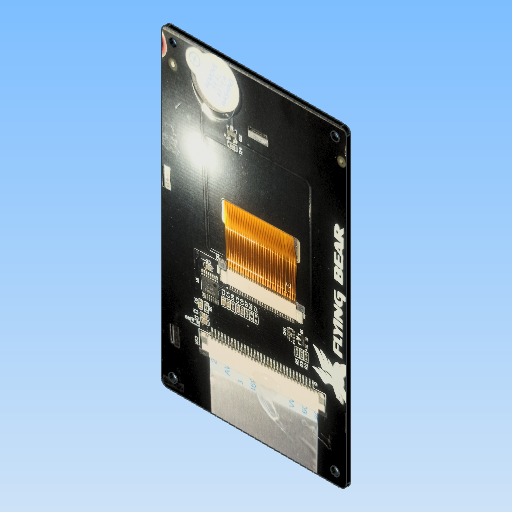
# Autodesk Inventor part: ЭКРАН
Saved by Autodesk Inventor 2017 (Build 210142000, 142)
## iProperties
Part Number: ЭКРАН
Material: Типовые
Document SubType Name: Modeling
Designer: Max
Mass: 9.96561 g
Surface Area: 147.746 cm^2
Volume: 9.96561 cm^3
Density: 1 g/cm^3
Appearance: Оружейный металл — полированный
Author: Max
Autodesk Inventor part; units mm, degrees
ref_plane "YZ Plane" through (0, 0, 0) normal (1, 0, 0) x (0, 1, 0)
ref_plane "XZ Plane" through (0, 0, 0) normal (0, 1, 0) x (-1, 0, 0)
ref_plane "XY Plane" through (0, 0, 0) normal (0, 0, 1) x (1, 0, 0)
sketch "Эскиз1" plane through (0, 0, 0) normal (0, 0, 1) x (1, 0, 0)
  line L0 (28.5, 51) -> (-28.5, 51) construction
  line L1 (-28.5, 51) -> (-28.5, -51) construction
  line L2 (-28.5, -51) -> (28.5, -51) construction
  line L3 (28.5, -51) -> (28.5, 51) construction
  line L4 (28.5, 51) -> (-28.5, -51) construction
  line L5 (-28.5, 51) -> (28.5, -51) construction
  circle A0 centre (-28.5, 51) radius 1.5
  circle A1 centre (28.5, 51) radius 1.5
  circle A2 centre (-28.5, -51) radius 1.5
  circle A3 centre (28.5, -51) radius 1.5
  line L6 (32.5, -55) -> (-32.5, -55)
  line L7 (-32.5, -55) -> (-32.5, 55)
  line L8 (-32.5, 55) -> (32.5, 55)
  line L9 (32.5, 55) -> (32.5, -55)
  line L10 (32.5, -55) -> (-32.5, 55) construction
  line L11 (-32.5, -55) -> (32.5, 55) construction
  point P0 (0, 0)
  point P1 (0, 0)
  dimension "d0" = 57
  dimension "d1" = 102
  dimension "d2" = 3
  dimension "d3" = 3
  dimension "d4" = 3
  dimension "d5" = 3
  dimension "d6" = 65
  dimension "d7" = 110
  constraints: 24 end point, 6 midpoint, 4 centre point, 4 coincident, 4 parallel, 2 horizontal, 2 perpendicular
  measures "d0" distance of L2.end L1.end
  measures "d1" distance of L1.end L0.end
  measures "d2" diameter of A0
  measures "d3" diameter of A1
  measures "d4" diameter of A2
  measures "d5" diameter of A3
  measures "d6" distance between parallel lines of L9 L7
  measures "d7" distance between parallel lines of L6 L8
extrude "Выдавливание1" add sketch "Эскиз1" along normal blind 1.4
fillet "Сопряжение1" radius 2 4 edges at (-32.5, 55, 0.7) (32.5, 55, 0.7) (-32.5, -55, 0.7) (32.5, -55, 0.7)
sketch "Эскиз2" plane through (0, 0, 1.4) normal (0, 0, 1) x (1, 0, 0)
  line L0 (36.1838, 87.7862) -> (49.9544, -99.5548) construction
  line L1 (49.9544, -99.5548) -> (-36.5855, -105.916) construction
  line L2 (-36.5855, -105.916) -> (-50.3561, 81.4251) construction
  line L3 (-50.3561, 81.4251) -> (36.1838, 87.7862) construction
  arc A0 (30.5, -55) -> (32.5, -53) centre (30.5, -53) ccw projected
  line L4 (32.5, -53) -> (32.5, 53) projected
  arc A1 (32.5, 53) -> (30.5, 55) centre (30.5, 53) ccw projected
  line L5 (30.5, 55) -> (-30.5, 55) projected
  arc A2 (-30.5, 55) -> (-32.5, 53) centre (-30.5, 53) ccw projected
  line L6 (-32.5, 53) -> (-32.5, -53) projected
  arc A3 (-32.5, -53) -> (-30.5, -55) centre (-30.5, -53) ccw projected
  line L7 (-30.5, -55) -> (30.5, -55) projected
  circle A4 centre (28.5, -51) radius 1.5 projected
  circle A5 centre (-28.5, -51) radius 1.5 projected
  circle A6 centre (28.5, 51) radius 1.5 projected
  circle A7 centre (-28.5, 51) radius 1.5 projected
  point P0 (0, 0)
  constraints: 2 other
decal "Маркировка1"
sketch "Эскиз3" plane through (0, 0, 0) normal (0, 0, -1) x (-1, 0, 0)
  line L0 (-24.5, 37) -> (24.5, 37) projected
  line L1 (24.5, 37) -> (24.5, -37) projected
  line L2 (24.5, -37) -> (-24.5, -37) projected
  line L3 (-24.5, -37) -> (-24.5, 37) projected
  ellipse E0 centre (-33.2228, -110.0838) end of major axis (-36.8911, -105.1818) minor radius 4 (-35.1117, -104.6274) -> (-36, -104.7456) ccw projected
  line L4 (34.1288, -104.6274) -> (-35.1117, -104.6274) projected
  ellipse E1 centre (30.2103, -110.0838) end of major axis (36.8811, -105.7867) minor radius 4 (35.9716, -104.9988) -> (34.1288, -104.6274) ccw projected
  line L5 (35.9716, 104.9988) -> (35.9716, -104.9988) projected
  ellipse E2 centre (30.2103, 110.0838) end of major axis (36.8811, 105.7867) minor radius 4 (34.1288, 104.6274) -> (35.9716, 104.9988) ccw projected
  line L6 (-35.1117, 104.6274) -> (34.1288, 104.6274) projected
  ellipse E3 centre (-33.2228, 110.0838) end of major axis (-36.8911, 105.1818) minor radius 4 (-36, 104.7456) -> (-35.1117, 104.6274) ccw projected
  line L7 (-36, -104.7456) -> (-36, 104.7456) projected
  line L8 (69.7943, 59.0707) -> (69.7943, -58.9868) construction
  line L9 (69.7943, -58.9868) -> (-33.2981, -58.9868) construction
  line L10 (-33.2981, -58.9868) -> (-33.2981, 59.0707) construction
  line L11 (-33.2981, 59.0707) -> (69.7943, 59.0707) construction
  point P0 (0, 0)
  constraints: 6 other
decal "Маркировка2"
